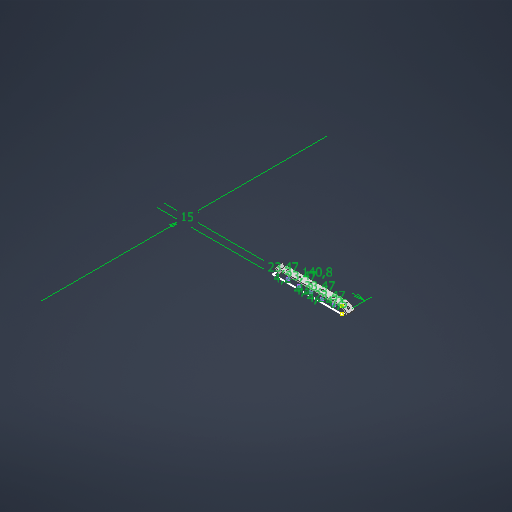
# Autodesk Inventor part: для жгутов2 ipt
Saved by Autodesk Inventor 2026.2 (Build 302298000, 298)
## iProperties
Created: 2026-01-08
Part Number: для жгутов2 ipt
Material: Типовые
Document SubType Name: Modeling
Designer: Phantom_HP2
Density: 1 g/cm^3
Appearance: По умолчанию
Author: Phantom_HP2
Autodesk Inventor part; units mm, degrees
ref_plane "YZ Plane" through (0, 0, 0) normal (1, 0, 0) x (0, 1, 0)
ref_plane "XZ Plane" through (0, 0, 0) normal (0, 1, 0) x (-1, 0, 0)
ref_plane "XY Plane" through (0, 0, 0) normal (0, 0, 1) x (1, 0, 0)
sketch "Эскиз1" plane through (0, 0, 0) normal (0, 1, 0) x (-1, 0, 0)
  line L0 (0, 0) -> (140.8, 0)
  line L1 (140.8, 0) -> (140.8, -15)
  line L2 (140.8, -15) -> (0, -15)
  circle A0 centre (23.47, -7.5) radius 2.1
  circle A1 centre (46.94, -7.5) radius 2.1
  circle A2 centre (70.41, -7.5) radius 2.1
  circle A3 centre (93.86, -7.5) radius 2.1
  circle A4 centre (117.33, -7.5) radius 2.1
  line L3 (0, 0) -> (0, -15)
  dimension "d1" = 15
  dimension "d2" = 140.8
  dimension "d3" = 4.2
  dimension "d5" = 7.5
  dimension "d6" = 4.2
  dimension "d8" = 4.2
  dimension "d10" = 4.2
  dimension "d12" = 4.2
  dimension "d14" = 23.47
  dimension "d16" = 23.47
  dimension "d17" = 23.47
  dimension "d18" = 23.47
  constraints: 8 end point, 5 centre point, 1 horizontal, 1 parallel, 1 perpendicular, 1 vertical
  measures "d1" distance of L0.end L1.end
  measures "d2" distance of L1.end L2.end
  measures "d3" diameter of A0
  measures "d5" distance from line of L2 A0.centre
  measures "d6" diameter of A1
  measures "d8" diameter of A2
  measures "d10" diameter of A3
  measures "d12" diameter of A4
  measures "d14" distance from line of L1 A4.centre
  measures "d16" distance of A1.centre A0.centre
  measures "d17" distance of A4.centre A3.centre
  measures "d18" distance of A1.centre A2.centre
extrude "Выдавливание1" add sketch "Эскиз1" along normal blind 15
sketch "Эскиз5" plane through (0, 0, -15) normal (0, 0, -1) x (-1, 0, 0)
  line L0 (0, 0) -> (140.8, 0) projected
  line L1 (140.8, 0) -> (140.8, 15) projected
  line L2 (0, 15) -> (140.8, 15) projected
  line L3 (0, 0) -> (0, 15) projected
  line L4 (0, 0) -> (0, 15) projected
  line L5 (-19.0591, -3.0798) -> (-12.1964, -13.0798)
  line L6 (-12.1964, -13.0798) -> (6.8628, 0)
  line L7 (0, 15) -> (-21.3918, 0.3193)
  line L8 (-19.0591, -3.0798) -> (-21.3918, 0.3193)
  line L9 (0, 15) -> (6.8628, 0)
  dimension "d63" = 10
  constraints: 10 end point, 2 perpendicular, 1 point on line
  measures "d63" vertical distance of L5.start L5.end
extrude "Выдавливание4" add sketch "Эскиз5" against normal blind 15 contours L0 L6 L5 L8 L7 L3 | L9 L2 L1 L0
sketch "Эскиз7" plane through (-140.8, 0, -15) normal (0, 0, -1) x (-1, 0, 0)
  line L0 (-155.8, -0.8981) -> (-138.4224, 11.7275) projected
  line L1 (-140.8, 15) -> (-93.6153, -51.5286)
  line L2 (-93.6153, -51.5286) -> (0.1874, 15)
  line L3 (-140.8, 15) -> (0, 15) projected
  line L4 (-20.962, 0) -> (0, 0)
  line L5 (0, 0) -> (0, 15)
  line L6 (-140.8, 15) -> (0, 15)
  line L7 (-20.962, 0) -> (0, 0)
  line L8 (0.1874, 15) -> (0.1874, 0)
  line L9 (0, 0) -> (0, 15) projected
  point P0 (-140.8, 0)
  point P1 (0, 14.8671)
  dimension "d50" = 81.5625
  dimension "d51" = 115
  dimension "d52" = 0
  constraints: 14 end point, 3 perpendicular, 2 point on line, 1 collinear, 1 horizontal, 1 vertical, 1 other
  measures "d50" distance of L0.end L1.end
  measures "d51" distance of L1.end L2.end
  measures "d52" distance from line of L3 L2.end
extrude "Выдавливание6" cut sketch "Эскиз7" against normal blind 15 contours L5 L4 L2
sketch "Эскиз8" plane through (0, 15, -15) normal (0, 0, -1) x (-1, 0, 0)
  line L0 (0, 0) -> (140.8, 0) projected
  line L1 (0, 0) -> (36.7423, -59.5819)
  line L2 (36.7423, -59.5819) -> (123.5616, -6.0432)
  line L3 (0, 0) -> (-29.0636, -18.4877)
  circle A0 centre (123.5616, -6.0432) radius 2.1
  point P0 (0, -15)
  dimension "d55" = 70
  dimension "d56" = 102
  dimension "d76" = 4.2
  constraints: 6 end point, 1 centre point, 1 coincident, 1 perpendicular
  measures "d55" distance of L0.start L1.end
  measures "d56" distance of L1.end L2.end
  measures "d76" diameter of A0
sketch "Эскиз10" plane through (0, 15, 0) normal (0.5658425, 0.8245133, 0) x (0.8245133, -0.5658425, 0)
  circle A0 centre (18.4448, 7.5) radius 2.1
  line L0 (25.9448, 0) -> (0, 0) projected
  line L1 (25.9448, 15) -> (25.9448, 0) projected
  point P0 (8.4876, 0)
  dimension "d69" = 4.2
  dimension "d70" = 7.5
  dimension "d71" = 7.5
  constraints: 1 centre point
  measures "d69" diameter of A0
  measures "d70" distance from line of L0 A0.centre
  measures "d71" distance from line of L1 A0.centre
extrude "Выдавливание9" cut sketch "Эскиз10" against normal blind 15
sketch "Эскиз11" plane through (0, 15, 0) normal (0, 1, 0) x (1, 0, 0)
  point P0 (0, 0)
sketch "Эскиз12" plane through (0, 15, 0) normal (0, 1, 0) x (1, 0, 0)
  circle A0 centre (-23.47, 7.5) radius 2.1 projected
  circle A1 centre (-46.94, 7.5) radius 2.1 projected
  circle A2 centre (-70.41, 7.5) radius 2.1 projected
  circle A3 centre (-93.86, 7.5) radius 2.1 projected
  circle A4 centre (-117.33, 7.5) radius 2.1 projected
  point P0 (0, 0)
extrude "Выдавливание10" cut sketch "Эскиз12" against normal blind 15
extrude "Выдавливание11" cut sketch "Эскиз8" against normal blind 15
sketch "Эскиз13" plane through (-140.8, 15, 0) normal (0, 0, 1) x (1, 0, 0)
  point P0 (140.8, -15)
sketch "Эскиз14" plane through (-140.8, 15, 0) normal (0, 0, 1) x (1, 0, 0)
  line L0 (140.8, 0) -> (0, 0) projected
  line L1 (0, 0) -> (-37, 0)
  line L2 (-37, 0) -> (-15.8506, -15)
  line L3 (-15.8506, -15) -> (6.9783, -15)
  line L4 (0, -0.1329) -> (20.962, -15) projected
  line L5 (0, -0.1329) -> (20.962, -15)
  line L6 (6.9783, -15) -> (20.962, -15)
  point P0 (140.8, -15)
  dimension "d79" = 37
  constraints: 10 end point, 2 horizontal, 2 parallel, 1 collinear, 1 point on line
  measures "d79" distance of L0.end L1.end
extrude "Выдавливание12" add sketch "Эскиз14" against normal blind 15 fills toward (70.4, -0.05) open curves L0 L1 L2 L3 L6
sketch "Эскиз15" plane through (-177.8, 15, 0) normal (0, 0, 1) x (1, 0, 0)
  line L0 (199.1918, -14.6807) -> (189.9964, -28.0798) projected
  line L1 (196.7887, -18.1824) -> (176.257, -4.092)
  line L2 (176.257, -4.092) -> (-2.2045, -2.6356)
  line L3 (-2.2045, -2.6356) -> (22.7303, -26.1279)
  line L4 (22.7303, -26.1279) -> (189.9964, -36.2255)
  line L5 (189.9964, -36.2255) -> (196.7887, -18.1824)
  point P0 (177.8, -15)
  constraints: 10 end point, 1 perpendicular, 1 point on line
extrude "Выдавливание13" cut sketch "Эскиз15" against normal blind 8
sketch "Эскиз16" plane through (-177.8, 15, -8) normal (0, 0, 1) x (1, 0, 0)
  point P0 (177.8, -15)
sketch "Эскиз17" plane through (-177.8, 15, -8) normal (0, 0, 1) x (1, 0, 0)
  line L0 (3.7851, -2.6845) -> (176.257, -4.092) projected
  line L1 (176.257, -4.092) -> (188.9232, -12.7845) projected
  line L2 (3.7851, -2.6845) -> (176.257, -4.092)
  line L3 (176.257, -4.092) -> (214.4439, -30.2987)
  line L4 (214.4439, -30.2987) -> (97.3846, -64.0666)
  line L5 (97.3846, -64.0666) -> (-1.4773, -35.1954)
  line L6 (-1.4773, -35.1954) -> (3.7851, -2.6845)
  point P0 (177.8, -15)
  constraints: 10 end point, 1 collinear
extrude "Выдавливание14" cut sketch "Эскиз17" against normal blind 8
sketch "Эскиз18" plane through (-177.8, 15, 0) normal (0, 0, 1) x (1, 0, 0)
  line L0 (177.8, 0) -> (199.1918, -14.6807) projected
  line L1 (177.8, 0) -> (176.257, -4.092)
  line L2 (176.257, -4.092) -> (193.5103, -30.0978)
  line L3 (193.5103, -30.0978) -> (209.0736, -14.129)
  line L4 (209.0736, -14.129) -> (177.8, 0)
  point P0 (177.8, -15)
  constraints: 8 end point
extrude "Выдавливание15" cut sketch "Эскиз18" against normal blind 15
sketch "Эскиз21" plane through (-177.8, 15, 0) normal (0, 0, 1) x (1, 0, 0)
  line L0 (177.8, 0) -> (0, 0) projected
  line L1 (177.8, 0) -> (189.9353, -8.8168)
  line L2 (177.8, 0) -> (176.257, -4.092) projected
  line L3 (176.257, -4.092) -> (187.4563, -12.2288)
  line L4 (189.9353, -8.8168) -> (187.4563, -12.2288)
  point P0 (177.8, -15)
  dimension "d92" = 15
  dimension "d94" = 36
  constraints: 6 end point, 1 parallel, 1 perpendicular
  measures "d92" distance of L0.start L1.end
  measures "d94" angle of L0 L1
extrude "Выдавливание17" add sketch "Эскиз21" against normal blind 15
sketch "Эскиз22" plane through (12.1353, 6.1832, 0) normal (0.5877853, 0.809017, 0) x (0.809017, -0.5877853, 0)
  circle A0 centre (-7.5, 7.5) radius 2.1
  line L0 (-15, 15) -> (0, 15) projected
  line L1 (0, 0) -> (0, 15) projected
  point P0 (-6.1832, 0)
  dimension "d97" = 4.2
  dimension "d98" = 7.5
  dimension "d99" = 7.5
  constraints: 1 centre point
  measures "d97" diameter of A0
  measures "d98" distance from line of L0 A0.centre
  measures "d99" distance from line of L1 A0.centre
extrude "Выдавливание18" cut sketch "Эскиз22" against normal blind 15
sketch "Эскиз23" plane through (-177.8, 15, 0) normal (0, 0, 1) x (1, 0, 0)
  line L0 (189.9353, -8.8168) -> (177.8, 0) projected
  line L1 (186.549, -103.0788) -> (-44.6132, 64.8703)
  line L2 (-44.6132, 64.8703) -> (-26.2742, -77.5538)
  line L3 (-26.2742, -77.5538) -> (186.549, -103.0788)
  point P0 (177.8, -15)
  dimension "d106" = 78.25
  constraints: 6 end point, 1 parallel
  measures "d106" distance between parallel lines of L0 L1
extrude "Выдавливание19" cut sketch "Эскиз23" against normal blind 15
sketch "Эскиз24" plane through (-133.1269, 15, 0) normal (0, 0, 1) x (1, 0, 0)
  line L0 (133.1269, 0) -> (0, 0) projected
  line L1 (12.3018, 0) -> (7.7798, -5.6524)
  line L2 (4.2014, -3.0525) -> (131.5839, -4.092) projected
  line L3 (0, 0) -> (4.2014, -3.0525) projected
  line L4 (0, 0) -> (7.7798, -5.6524)
  line L5 (12.3018, 0) -> (9.3018, 0)
  line L6 (0, 0) -> (3, 0)
  line L7 (145.2621, -8.8168) -> (133.1269, 0) projected
  line L8 (12.3018, 0) -> (0, 0)
  point P0 (133.1269, -15)
  constraints: 10 end point, 3 point on line, 2 collinear, 1 parallel
extrude "Выдавливание20" cut sketch "Эскиз24" against normal blind 15
sketch "Эскиз25" plane through (-120.8251, 15, 0) normal (0, 0, 1) x (1, 0, 0)
  line L0 (120.8251, 0) -> (0, 0) projected
  line L1 (0, 0) -> (-7.231, -9.9526)
  line L2 (-7.231, -9.9526) -> (-17.231, -2.6872)
  line L3 (132.9603, -8.8168) -> (120.8251, 0) projected
  line L4 (-17.231, -2.6872) -> (-14.8799, 0.5489)
  line L5 (-14.8799, 0.5489) -> (-8.8799, -3.8363)
  line L6 (-8.8799, -3.8363) -> (-6.0761, 0)
  line L7 (-6.0761, 0) -> (0, 0)
  point P0 (120.8251, -15)
  dimension "d113" = 7.231
  dimension "d114" = 10
  dimension "d115" = 4
  dimension "d117" = 6
  constraints: 12 end point, 2 parallel, 2 perpendicular, 1 horizontal
  measures "d113" horizontal distance of L0.end L1.end
  measures "d114" horizontal distance of L1.end L2.end
  measures "d115" distance of L2.end L4.end
  measures "d117" horizontal distance of L4.end L5.end
extrude "Выдавливание21" add sketch "Эскиз25" against normal blind 15
